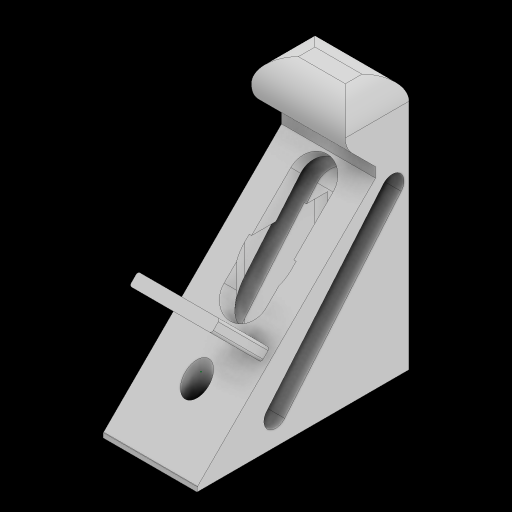
# Autodesk Inventor part: podstawka
Saved by Autodesk Inventor 2024.4 (Build 284460000, 460)
## iProperties
Created: 2025-10-11
Part Number: podstawka
Material: Ogólny
Document SubType Name: Modeling
Designer: User
Density: 1 g/cm^3
Appearance: Domyślna
Author: User
Autodesk Inventor part; units mm, degrees
ref_plane "YZ Plane" through (0, 0, 0) normal (1, 0, 0) x (0, 1, 0)
ref_plane "XZ Plane" through (0, 0, 0) normal (0, 1, 0) x (-1, 0, 0)
ref_plane "XY Plane" through (0, 0, 0) normal (0, 0, 1) x (1, 0, 0)
sketch "Szkic1" plane through (0, 0, 0) normal (0, 1, 0) x (-1, 0, 0)
  line L0 (-20, 45) -> (20, 45)
  line L1 (20, 45) -> (20, -45)
  line L2 (20, -45) -> (-20, -45)
  line L3 (-20, -45) -> (-20, 45)
  line L4 (-20, 45) -> (20, -45) construction
  line L5 (20, 45) -> (-20, -45) construction
  line L6 (0, 45) -> (0, 30)
  circle A0 centre (0, 30) radius 2
  point P0 (0, 0)
  dimension "d0" = 40
  dimension "d1" = 90
  dimension "d2" = 15
  dimension "d3" = 4
  constraints: 14 end point, 3 midpoint, 2 parallel, 1 centre point, 1 coincident, 1 horizontal, 1 perpendicular, 1 vertical
  measures "d0" distance of L1.end L2.end
  measures "d1" distance of L0.end L1.end
  measures "d2" distance of L6.start L6.end
  measures "d3" diameter of A0
extrude "Wyciągnięcie proste1" add sketch "Szkic1" along normal blind 2 contours L0 L1 L2 L3 | A0
sketch "Szkic2" plane through (20, 0, 45) normal (1, 0, 0) x (0, 0, -1)
  line L0 (0, 2) -> (90, 2) projected
  line L1 (0, 2) -> (90, 92)
  line L2 (0, 2) -> (127.2792, 2) construction
  line L3 (90, 92) -> (90, 2)
  line L4 (90, 92) -> (79.3934, 81.3934)
  line L5 (79.3934, 81.3934) -> (68.7868, 92)
  line L6 (68.7868, 92) -> (90, 92)
  point P0 (45, 0)
  dimension "d6" = 45
  dimension "d7" = 15
  constraints: 12 end point, 3 perpendicular, 1 equal length, 1 horizontal, 1 point on line
  measures "d6" angle of L2 L1
  measures "d7" distance of L1.end L4.end
extrude "Wyciągnięcie proste2" add sketch "Szkic2" against normal up to surface (40 mm away)
ref_plane "Płaszczyzna konstrukcyjna1" through (0, 0, 45) normal (1, 0, 0) x (0, 0, -1)
sketch "Szkic3" plane through (0, 0, 45) normal (1, 0, 0) x (0, 0, -1)
  line L0 (79.3934, 81.3934) -> (0, 2) projected
  line L1 (0, 2) -> (29.6985, 31.6985)
  line L2 (29.6985, 31.6985) -> (8.4853, 52.9117)
  line L3 (8.4853, 52.9117) -> (12.0208, 56.4472)
  line L4 (12.0208, 56.4472) -> (33.234, 35.234)
  line L5 (33.234, 35.234) -> (29.6985, 31.6985)
  point P0 (45, 0)
  dimension "d11" = 42
  dimension "d12" = 30
  dimension "d13" = 5
  dimension "d14" = 90
  constraints: 10 end point, 2 perpendicular, 2 point on line, 1 collinear
  measures "d11" distance of L0.end L1.end
  measures "d12" distance of L1.end L2.end
  measures "d13" distance of L2.end L3.end
  measures "d14" angle of L3 L4
extrude "Wyciągnięcie proste3" add sketch "Szkic3" along normal mid plane 35
sketch "Szkic4" plane through (0, 0, 0) normal (0, -1, 0) x (1, 0, 0)
  line L0 (-20, 45) -> (20, 45) projected
  line L1 (0, 45) -> (0, 47)
  line L2 (0, 47) -> (0, 67)
  circle A0 centre (0, 47) radius 2
  line L3 (20, 45) -> (-20, 45)
  line L4 (-20, 45) -> (-20, 67)
  line L5 (-20, 67) -> (20, 67)
  line L6 (20, 67) -> (20, 45)
  point P0 (0, 0)
  dimension "d17" = 2
  dimension "d18" = 20
  dimension "d19" = 4
  dimension "d20" = 40
  dimension "d22" = 0
  constraints: 12 end point, 2 parallel, 2 vertical, 1 centre point, 1 coincident, 1 horizontal, 1 midpoint, 1 perpendicular
  measures "d17" distance of L1.start L1.end
  measures "d18" distance of L1.end L2.end
  measures "d19" diameter of A0
  measures "d20" distance of L4.end L5.end
  measures "d22" distance from line of L2.end L5
extrude "Wyciągnięcie proste4" add sketch "Szkic4" against normal blind 2 contours L4 L5 L2 A0 L0 | A0 L2 L5 L6 L0
sketch "Szkic5" plane through (-20, 81.3934, -34.3934) normal (0, 0.7071068, 0.7071068) x (1, 0, 0)
  point P0 (20, -81.8736)
move faces "Przesuń1" translate (0, 17, 20) faces at (6.6667, 92, -37.9289) (6.6667, 88.4645, -27.3223)
chamfer "Faza1" distance 3 angle 45 1 edges at (0, 79.8934, -32.8934)
fillet "Zaokrąglenie1" radius 1 4 edges at (17.5, 45.8406, 22.3726) (17.5, 42.3051, 25.9081) (-17.5, 42.3051, 25.9081) (-17.5, 45.8406, 22.3726)
fillet "Zaokrąglenie3" radius 10 4 edges at (0, 109, -45) (-20, 109, -24.3934) (20, 109, -24.3934) (0, 109, -3.7868)
sketch "Szkic6" plane through (-20, 2, 45) normal (0, 0.7071068, 0.7071068) x (1, 0, 0)
  line L0 (0, 107.1579) -> (40, 107.1579) projected
  line L1 (20, 107.1579) -> (20, 97.1579)
  line L2 (3.5, 47) -> (36.5, 47) projected
  line L3 (20, 47) -> (20, 57)
  line L4 (20, 57) -> (20, 97.1579) construction
  line L5 (29, 57) -> (29, 97.1579)
  line L6 (11, 97.1579) -> (11, 57)
  arc A0 (11, 57) -> (29, 57) centre (20, 57) ccw
  arc A1 (29, 97.1579) -> (11, 97.1579) centre (20, 97.1579) ccw
  point P0 (20, 30.4056)
  point P1 (20, 77.079)
  dimension "d34" = 10
  dimension "d35" = 10
  dimension "d36" = 18
  constraints: 12 end point, 4 point on circle, 4 tangent, 3 midpoint, 3 vertical, 2 centre point, 1 parallel
  measures "d34" distance of L1.start L1.end
  measures "d35" distance of L3.start L3.end
  measures "d36" diameter of A1
extrude "Wyciągnięcie proste5" cut sketch "Szkic6" against normal blind 84
sketch "Szkic7" plane through (0, 0, 0) normal (0, -1, 0) x (1, 0, 0)
  line L0 (9, -45) -> (-9, -45) projected
  line L1 (0, -45) -> (0, -35)
  line L2 (-10, -35) -> (10, -35) projected
  line L3 (-20, 45) -> (0, 45) projected
  line L4 (0, 45) -> (0, -5)
  line L5 (0, -5) -> (0, -35) construction
  line L6 (-10, -5) -> (-10, -35)
  line L7 (10, -35) -> (10, -5)
  arc A0 (10, -5) -> (-10, -5) centre (0, -5) ccw
  arc A1 (-10, -35) -> (10, -35) centre (0, -35) ccw
  point P0 (0, 0)
  point P1 (0, -20)
  point P2 (10, -35)
  dimension "d39" = 10
  dimension "d40" = 50
  dimension "d41" = 20
  constraints: 12 end point, 4 point on circle, 4 tangent, 3 midpoint, 2 centre point, 1 collinear, 1 parallel, 1 vertical
  measures "d39" distance of L1.start L1.end
  measures "d40" distance of L3.end L4.end
  measures "d41" diameter of A1
extrude "Wyciągnięcie proste6" cut sketch "Szkic7" against normal blind 54
sketch "Szkic8" plane through (20, 0, 67) normal (1, 0, 0) x (0, 0, -1)
  line L0 (97.7721, 77.7721) -> (22, 2) projected
  line L1 (43.5, 23.5) -> (67, 0)
  line L2 (97.7721, 77.7721) -> (112, 63.5442)
  line L3 (112, 0) -> (112, 99) projected
  line L4 (55.25, 11.75) -> (104.886, 70.6581) construction
  line L5 (59.0736, 8.5282) -> (108.7097, 67.4363)
  line L6 (101.0624, 73.8799) -> (51.4264, 14.9718)
  arc A0 (51.4264, 14.9718) -> (59.0736, 8.5282) centre (55.25, 11.75) ccw
  arc A1 (108.7097, 67.4363) -> (101.0624, 73.8799) centre (104.886, 70.6581) ccw
  point P0 (80.068, 41.2041)
  dimension "d44" = 10
  constraints: 12 end point, 4 point on circle, 4 tangent, 3 midpoint, 2 centre point, 2 point on line, 1 parallel, 1 perpendicular
  measures "d44" diameter of A1
extrude "Wyciągnięcie proste7" cut sketch "Szkic8" against normal blind 86.5 contours A1 L5 L2 | L2 L5 A0 L1 L6 A1 | L1 A0 L6
move faces "Przesuń2" translate (0, 0, -21.75) faces at (-0.2453, 1.3333, 45.0151) (6.6667, 0.6667, 67)
sketch "Szkic9" plane through (0, 0, 0) normal (0, -1, 0) x (1, 0, 0)
  circle A0 centre (0, 25.25) radius 2 projected
  circle A1 centre (0, 25.25) radius 2
  point P0 (0, 0)
  constraints: 1 centre point, 1 coincident
extrude "Wyciągnięcie proste8" cut sketch "Szkic9" against normal blind 37.25
ref_plane "Płaszczyzna konstrukcyjna2" through (0, 3, 0) normal (0, -1, 0) x (1, 0, 0)
sketch "Szkic10" plane through (0, 3, 0) normal (0, -1, 0) x (1, 0, 0)
  circle A0 centre (0, 25.25) radius 2 projected
  circle A1 centre (0, 25.25) radius 5
  point P0 (0, 0)
  dimension "d56" = 10
  constraints: 1 centre point, 1 coincident
  measures "d56" diameter of A1
extrude "Wyciągnięcie proste9" cut sketch "Szkic10" against normal blind 56 contours A0 | A1
